# Autodesk Inventor part: NPN_SM
Saved by Autodesk Inventor 2015 SP1 (Build 190203100, 203)
## iProperties
Created: 2015-06-25
Part Number: NPN_SM
Material: Generic
Document SubType Name: Modeling
Designer: Patrick
Density: 1 g/cm^3
Appearance: SOT23, NPN_SM
Author: Patrick
Autodesk Inventor part; units mm, degrees
ref_plane "YZ Plane" through (0, 0, 0) normal (1, 0, 0) x (0, 1, 0)
ref_plane "XZ Plane" through (0, 0, 0) normal (0, 1, 0) x (-1, 0, 0)
ref_plane "XY Plane" through (0, 0, 0) normal (0, 0, 1) x (1, 0, 0)
sketch "SOT23, NPN_SM_154" plane through (0, 0, 0) normal (0, 0, 1) x (1, 0, 0)
  line L0 (-1.715, -1.55) -> (-1.715, 2.014)
  line L1 (-1.715, 2.014) -> (1.715, 2.014)
  line L2 (1.715, 2.014) -> (1.715, -1.55)
  line L3 (1.715, -1.55) -> (-1.715, -1.55)
  constraints: 8 end point
extrude "Extrusion1" add sketch "SOT23, NPN_SM_154" along normal blind 1
body "Solid1"
